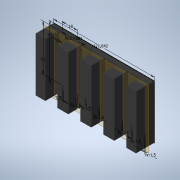
# Autodesk Inventor part: LinearRegulator_Fixation
Saved by Autodesk Inventor 2022 (Build 260153000, 153)
## iProperties
Created: 2023-08-16
Part Number: LinearRegulator_Fixation
Material: Generisch
Document SubType Name: Modeling
Designer: aewalder
Mass: 127.682 g
Surface Area: 346.921 cm^2
Volume: 127.682 cm^3
Density: 1 g/cm^3
Appearance: Vorgabe
Author: aewalder
Autodesk Inventor part; units mm, degrees
ref_plane "YZ Plane" through (0, 0, 0) normal (1, 0, 0) x (0, 1, 0)
ref_plane "XZ Plane" through (0, 0, 0) normal (0, 1, 0) x (-1, 0, 0)
ref_plane "XY Plane" through (0, 0, 0) normal (0, 0, 1) x (1, 0, 0)
sketch "Sketch1" plane through (0, 0, 0) normal (0, 0, 1) x (1, 0, 0)
  line L0 (-60.8211, 32.5) -> (60.8211, 32.5)
  line L1 (60.8211, 32.5) -> (60.8211, -32.5)
  line L2 (60.8211, -32.5) -> (-60.8211, -32.5)
  line L3 (-60.8211, -32.5) -> (-60.8211, 32.5)
  line L4 (-60.8211, 32.5) -> (60.8211, -32.5) construction
  line L5 (60.8211, 32.5) -> (-60.8211, -32.5) construction
  line L6 (-60.8211, 0) -> (60.8211, 0) construction
  line L7 (-50.8211, 28) -> (-32.8211, 28) construction
  line L8 (-32.8211, 28) -> (-32.8211, -28) construction
  line L9 (-32.8211, -28) -> (-50.8211, -28) construction
  line L10 (-50.8211, -28) -> (-50.8211, 28) construction
  line L11 (-50.8211, 28) -> (-32.8211, -28) construction
  line L12 (-32.8211, 28) -> (-50.8211, -28) construction
  line L13 (-22.9404, 28) -> (-4.9404, 28) construction
  line L14 (-4.9404, 28) -> (-4.9404, -28) construction
  line L15 (-4.9404, -28) -> (-22.9404, -28) construction
  line L16 (-22.9404, -28) -> (-22.9404, 28) construction
  line L17 (-22.9404, 28) -> (-4.9404, -28) construction
  line L18 (-4.9404, 28) -> (-22.9404, -28) construction
  line L19 (4.9404, 28) -> (22.9404, 28) construction
  line L20 (22.9404, 28) -> (22.9404, -28) construction
  line L21 (22.9404, -28) -> (4.9404, -28) construction
  line L22 (4.9404, -28) -> (4.9404, 28) construction
  line L23 (4.9404, 28) -> (22.9404, -28) construction
  line L24 (22.9404, 28) -> (4.9404, -28) construction
  line L25 (32.8211, 28) -> (50.8211, 28) construction
  line L26 (50.8211, 28) -> (50.8211, -28) construction
  line L27 (50.8211, -28) -> (32.8211, -28) construction
  line L28 (32.8211, -28) -> (32.8211, 28) construction
  line L29 (32.8211, 28) -> (50.8211, -28) construction
  line L30 (50.8211, 28) -> (32.8211, -28) construction
  line L31 (-60.8211, 32.5) -> (-49.3211, 32.5)
  line L32 (-49.3211, 32.5) -> (-49.3211, -32.5)
  line L33 (-49.3211, -32.5) -> (-60.8211, -32.5)
  line L34 (-60.8211, -32.5) -> (-60.8211, 32.5)
  line L35 (-34.3211, 32.5) -> (-21.4404, 32.5)
  line L36 (-21.4404, 32.5) -> (-21.4404, -32.5)
  line L37 (-21.4404, -32.5) -> (-34.3211, -32.5)
  line L38 (-34.3211, -32.5) -> (-34.3211, 32.5)
  line L39 (-34.3211, 32.5) -> (-21.4404, -32.5) construction
  line L40 (-21.4404, 32.5) -> (-34.3211, -32.5) construction
  line L41 (-6.4404, 32.5) -> (6.4404, 32.5)
  line L42 (6.4404, 32.5) -> (6.4404, -32.5)
  line L43 (6.4404, -32.5) -> (-6.4404, -32.5)
  line L44 (-6.4404, -32.5) -> (-6.4404, 32.5)
  line L45 (-6.4404, 32.5) -> (6.4404, -32.5) construction
  line L46 (6.4404, 32.5) -> (-6.4404, -32.5) construction
  line L47 (21.4404, 32.5) -> (34.3211, 32.5)
  line L48 (34.3211, 32.5) -> (34.3211, -32.5)
  line L49 (34.3211, -32.5) -> (21.4404, -32.5)
  line L50 (21.4404, -32.5) -> (21.4404, 32.5)
  line L51 (21.4404, 32.5) -> (34.3211, -32.5) construction
  line L52 (34.3211, 32.5) -> (21.4404, -32.5) construction
  line L53 (60.8211, 32.5) -> (49.3211, 32.5)
  line L54 (49.3211, 32.5) -> (49.3211, -32.5)
  line L55 (49.3211, -32.5) -> (60.8211, -32.5)
  line L56 (60.8211, -32.5) -> (60.8211, 32.5)
  line L57 (50.8211, 32.5) -> (50.8211, -32.5)
  line L58 (32.8211, -32.5) -> (32.8211, 32.5)
  line L59 (22.9404, 32.5) -> (22.9404, -32.5)
  line L60 (4.9404, -32.5) -> (4.9404, 32.5)
  line L61 (-4.9404, 32.5) -> (-4.9404, -32.5)
  line L62 (-22.9404, -32.5) -> (-22.9404, 32.5)
  line L63 (-32.8211, 32.5) -> (-32.8211, -32.5)
  line L64 (-50.8211, -32.5) -> (-50.8211, 32.5)
  point P0 (0, 0)
  point P1 (-41.8211, 0)
  point P2 (-13.9404, 0)
  point P3 (13.9404, 0)
  point P4 (41.8211, 0)
  point P5 (-27.8807, 0)
  point P6 (27.8807, 0)
  point P7 (-6.4404, -32.5)
  point P8 (6.4404, 32.5)
  point P9 (-50.8211, 32.5)
  point P10 (-32.8211, -32.5)
  point P11 (32.8211, 32.5)
  dimension "d0" = 18
  dimension "d1" = 56
  dimension "d2" = 121.6421
  dimension "d3" = 10
  dimension "d6" = 27.8807
  dimension "d11" = 65
  dimension "d12" = 1.5
  dimension "d13" = 1.5
  dimension "d14" = 1.5
  dimension "d15" = 1.5
  dimension "d16" = 1.5
  dimension "d17" = 1.5
  dimension "d18" = 1.5
  constraints: 130 end point, 31 point on line, 18 midpoint, 16 parallel, 9 collinear, 9 perpendicular, 8 horizontal, 33 other
  measures "d0" distance of L7.start L7.end
  measures "d1" distance between parallel lines of L9 L7
  measures "d2" distance of L0.start L0.end
  measures "d3" distance between parallel lines of L10 L3
  measures "d6" distance of L7.start L13.start
  measures "d11" distance of L2.end L0.start
  measures "d12" distance between parallel lines of L10 L32
  measures "d13" distance between parallel lines of L38 L8
  measures "d14" distance between parallel lines of L16 L36
  measures "d15" distance between parallel lines of L14 L44
  measures "d16" distance between parallel lines of L20 L50
  measures "d17" distance between parallel lines of L28 L48
  measures "d18" distance between parallel lines of L26 L54
extrude "Extrusion1" add sketch "Sketch1" along normal blind 5
extrude "Extrusion2" add sketch "Sketch1" along normal blind 17 from surface at 5 contours L0 L64 L2 L3 | L0 L32 L2 L64 | L0 L63 L2 L38 | L0 L62 L2 L63 | L0 L36 L2 L62 | L0 L61 L2 L44 | L0 L60 L2 L61 | L0 L42 L2 L60 | L0 L59 L2 L50 | L0 L58 L2 L59 | L0 L48 L2 L58 | L0 L57 L2 L54 | L0 L1 L2 L57
ref_plane "Work Plane1" through (0, 0, 11) normal (0, 0, 1) x (1, 0, 0)
extrude "Extrusion3" cut sketch "Sketch1" along normal mid plane 0.8 from surface at 11 contours L0 L32 L2 L64 | L0 L63 L2 L38 | L0 L36 L2 L62 | L0 L61 L2 L44 | L0 L42 L2 L60 | L0 L59 L2 L50 | L0 L48 L2 L58 | L0 L57 L2 L54
equation "\"d6\" = -0.333333 * d0 + 0.333333 * d2 - 0.666667 * d3"
equation "\"d13\" = d12"
equation "\"d14\" = d13"
equation "\"d15\" = d14"
equation "\"d16\" = d15"
equation "\"d17\" = d16"
equation "\"d18\" = d17"
body "Solid1"
